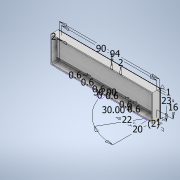
# Autodesk Inventor part: sdm_finger_eit_chamber_mould_horizontal_e_holes_v2
Saved by Autodesk Inventor 2021 (Build 250183000, 183)
## iProperties
Created: 2021-05-26
Part Number: sdm_finger_eit_chamber_mould_horizontal_e_holes_v2
Material: Generic
Document SubType Name: Modeling
Designer: Charlie
Density: 1 g/cm^3
Appearance: Default
Author: Charlie
Autodesk Inventor part; units mm, degrees
ref_plane "YZ Plane" through (0, 0, 0) normal (1, 0, 0) x (0, 1, 0)
ref_plane "XZ Plane" through (0, 0, 0) normal (0, 1, 0) x (-1, 0, 0)
ref_plane "XY Plane" through (0, 0, 0) normal (0, 0, 1) x (1, 0, 0)
sketch "Sketch2" plane through (0, 0, 0) normal (0, 0, 1) x (1, 0, 0)
  line L0 (-46, 11.5) -> (46, 11.5)
  line L1 (47, 10.5) -> (47, -10.5)
  line L2 (46, -11.5) -> (-46, -11.5)
  line L3 (-47, -10.5) -> (-47, 10.5)
  line L4 (-47, 11.5) -> (47, -11.5) construction
  line L5 (47, 11.5) -> (-47, -11.5) construction
  line L6 (48, 12.5) -> (-48, 12.5)
  line L7 (-48, 12.5) -> (-48, -12.5)
  line L8 (-48, -12.5) -> (48, -12.5)
  line L9 (48, -12.5) -> (48, 12.5)
  arc A0 (47, 10.5) -> (46, 11.5) centre (46, 10.5) ccw
  arc A1 (46, -11.5) -> (47, -10.5) centre (46, -10.5) ccw
  arc A2 (-47, -10.5) -> (-46, -11.5) centre (-46, -10.5) ccw
  arc A3 (-46, 11.5) -> (-47, 10.5) centre (-46, 10.5) ccw
  line L10 (-45, -6.5) -> (45, -6.5)
  line L11 (45, -6.5) -> (45, 9.5)
  line L12 (45, 9.5) -> (-45, 9.5)
  line L13 (-45, 9.5) -> (-45, -6.5)
  point P0 (0, 0)
  point P1 (0, 1.6851)
  dimension "d0" = 94
  dimension "d1" = 23
  dimension "d3" = 1
  dimension "d10" = 1
  dimension "d84" = 90
  dimension "d85" = 16
  dimension "d86" = 2
  dimension "d87" = 2
  dimension "d95" = 2
  constraints: 28 end point, 8 point on circle, 8 point on line, 8 tangent, 6 parallel, 4 centre point, 3 equal radius, 3 perpendicular, 2 horizontal, 2 midpoint, 3 other
  measures "d0" distance of L4.end L5.end
  measures "d1" distance of L5.start L4.end
  measures "d3" distance between parallel lines of L0 L6
  measures "d10" radius of A0
  measures "d84" distance of L12.end L11.end
  measures "d85" distance of L11.end L10.end
  measures "d86" distance between parallel lines of L0 L12
  measures "d87" distance between parallel lines of L3 L13
  measures "d95" distance between parallel lines of L1 L11
extrude "Extrusion1" add sketch "Sketch2" along normal blind 1 contours L0 A0 L1 A1 L2 A2 L3 A3 | L9 L8 L7 L6 | L13 L12 L11 L10
extrude "Extrusion2" add sketch "Sketch2" along normal blind 7 contours L9 L8 L7 L6
extrude "Extrusion3" add sketch "Sketch2" along normal blind 4 contours L13 L12 L11 L10
sketch "Sketch4" plane through (-48, -12.5, 0) normal (0, -1, 0) x (1, 0, 0)
  circle A0 centre (22.1132, 5) radius 0.5
  circle A1 centre (29.8868, 5) radius 0.5
  circle A2 centre (44.1132, 5) radius 0.5
  circle A3 centre (51.8842, 5) radius 0.5
  circle A4 centre (66.1132, 5) radius 0.5
  circle A5 centre (73.8868, 5) radius 0.5
  line L0 (0, 6) -> (96, 6)
  line L1 (96, 7) -> (0, 7) projected
  line L2 (22.1132, 2) -> (22.1132, 2)
  line L3 (22.6132, 2.5) -> (22.6132, 8)
  line L4 (22.6132, 8) -> (21.6132, 8)
  line L5 (21.6132, 8) -> (21.6132, 2.5)
  line L6 (21.6132, 2) -> (22.6132, 8) construction
  line L7 (22.6132, 2) -> (21.6132, 8) construction
  line L8 (29.8868, 2) -> (29.8868, 2)
  line L9 (30.3868, 2.5) -> (30.3868, 8)
  line L10 (30.3868, 8) -> (29.3868, 8)
  line L11 (29.3868, 8) -> (29.3868, 2.5)
  line L12 (29.3868, 2) -> (30.3868, 8) construction
  line L13 (30.3868, 2) -> (29.3868, 8) construction
  line L14 (44.1132, 2) -> (44.1132, 2)
  line L15 (44.6132, 2.5) -> (44.6132, 8)
  line L16 (44.6132, 8) -> (43.6132, 8)
  line L17 (43.6132, 8) -> (43.6132, 2.5)
  line L18 (43.6132, 2) -> (44.6132, 8) construction
  line L19 (44.6132, 2) -> (43.6132, 8) construction
  line L20 (51.8842, 2) -> (51.8842, 2)
  line L21 (52.3842, 2.5) -> (52.3842, 8)
  line L22 (52.3842, 8) -> (51.3842, 8)
  line L23 (51.3842, 8) -> (51.3842, 2.5)
  line L24 (51.3842, 2) -> (52.3842, 8) construction
  line L25 (52.3842, 2) -> (51.3842, 8) construction
  line L26 (66.1132, 2) -> (66.1132, 2)
  line L27 (65.6132, 2.5) -> (65.6132, 8)
  line L28 (65.6132, 8) -> (66.6132, 8)
  line L29 (66.6132, 8) -> (66.6132, 2.5)
  line L30 (66.6132, 2) -> (65.6132, 8) construction
  line L31 (65.6132, 2) -> (66.6132, 8) construction
  line L32 (73.8868, 2) -> (73.8868, 2)
  line L33 (73.3868, 2.5) -> (73.3868, 8)
  line L34 (73.3868, 8) -> (74.3868, 8)
  line L35 (74.3868, 8) -> (74.3868, 2.5)
  line L36 (74.3868, 2) -> (73.3868, 8) construction
  line L37 (73.3868, 2) -> (74.3868, 8) construction
  arc A6 (21.6132, 2.5) -> (22.1132, 2) centre (22.1132, 2.5) ccw
  arc A7 (22.1132, 2) -> (22.6132, 2.5) centre (22.1132, 2.5) ccw
  arc A8 (29.3868, 2.5) -> (29.8868, 2) centre (29.8868, 2.5) ccw
  arc A9 (29.8868, 2) -> (30.3868, 2.5) centre (29.8868, 2.5) ccw
  arc A10 (43.6132, 2.5) -> (44.1132, 2) centre (44.1132, 2.5) ccw
  arc A11 (44.1132, 2) -> (44.6132, 2.5) centre (44.1132, 2.5) ccw
  arc A12 (51.3842, 2.5) -> (51.8842, 2) centre (51.8842, 2.5) ccw
  arc A13 (51.8842, 2) -> (52.3842, 2.5) centre (51.8842, 2.5) ccw
  arc A14 (65.6132, 2.5) -> (66.1132, 2) centre (66.1132, 2.5) ccw
  arc A15 (66.1132, 2) -> (66.6132, 2.5) centre (66.1132, 2.5) ccw
  arc A16 (73.3868, 2.5) -> (73.8868, 2) centre (73.8868, 2.5) ccw
  arc A17 (73.8868, 2) -> (74.3868, 2.5) centre (73.8868, 2.5) ccw
  point P0 (96, 0)
  point P1 (69, 6)
  point P2 (71, 6)
  point P3 (49, 6)
  point P4 (47, 6)
  point P5 (27, 6)
  point P6 (25, 6)
  point P7 (73.8868, 2)
  point P8 (66.1132, 2)
  point P9 (51.8842, 2)
  point P10 (44.1132, 2)
  point P11 (29.8868, 2)
  point P12 (22.1132, 2)
  dimension "d59" = 1
  dimension "d60" = 1
  dimension "d61" = 1
  dimension "d62" = 1
  dimension "d63" = 1
  dimension "d64" = 1
  dimension "d65" = 1
  dimension "d66" = 6
  dimension "d67" = 1
  dimension "d68" = 6
  dimension "d69" = 1
  dimension "d70" = 6
  dimension "d71" = 1
  dimension "d72" = 6
  dimension "d73" = 1
  dimension "d74" = 6
  dimension "d75" = 1
  dimension "d76" = 6
  dimension "d81" = 0.5
  constraints: 74 end point, 24 point on circle, 24 point on line, 24 tangent, 18 centre point, 12 midpoint, 12 parallel, 11 equal radius, 6 horizontal, 6 perpendicular
  measures "d59" diameter of A0
  measures "d60" diameter of A1
  measures "d61" diameter of A2
  measures "d62" diameter of A3
  measures "d63" diameter of A4
  measures "d64" diameter of A5
  measures "d65" distance of L4.end L3.end
  measures "d66" distance of L3.end L7.start
  measures "d67" distance of L10.end L9.end
  measures "d68" distance of L9.end L13.start
  measures "d69" distance of L16.end L15.end
  measures "d70" distance of L15.end L19.start
  measures "d71" distance of L22.end L21.end
  measures "d72" distance of L21.end L25.start
  measures "d73" distance of L27.end L28.end
  measures "d74" distance of L31.start L27.end
  measures "d75" distance of L33.end L34.end
  measures "d76" distance of L37.start L33.end
  measures "d81" radius of A6
sketch "Sketch3" plane through (0, -12.5, 4) normal (0, -1, 0) x (1, 0, 0)
  line L0 (-53.1158, -2.5) -> (46.8842, -2.5) construction
  line L1 (43, -1.5) -> (23, -1.5) construction
  line L2 (23, -1.5) -> (23, 3.5) construction
  line L3 (23, 3.5) -> (43, 3.5) construction
  line L4 (43, 3.5) -> (43, -1.5) construction
  line L5 (23, -1.5) -> (23, 3.7137) construction
  line L6 (43, -1.5) -> (40.1132, 3.5) construction
  line L7 (46.8842, -2.5) -> (46.8842, 3.2735) construction
  line L8 (23, -1.5) -> (25.8868, 3.5) construction
  line L9 (23, -1.5) -> (23, 3.1279) construction
  line L10 (21, -1.5) -> (18.1132, 3.5) construction
  line L11 (1, 3.5) -> (21, 3.5) construction
  line L12 (1, -1.5) -> (3.8868, 3.5) construction
  line L13 (-1, -1.5) -> (-3.8868, 3.5) construction
  line L14 (-21, 3.5) -> (-1, 3.5) construction
  line L15 (-21, -1.5) -> (-18.1132, 3.5) construction
  line L16 (-23, -1.5) -> (-25.8868, 3.5) construction
  line L17 (-43, 3.5) -> (-23, 3.5) construction
  line L18 (-43, -1.5) -> (-40.1132, 3.5) construction
  line L19 (43, 3.5) -> (-43, 3.5) construction
  line L20 (0, 3.5) -> (0, 3.5) construction
  circle A0 centre (-25.8868, -1.5) radius 0.3
  circle A1 centre (-18.1132, -1.5) radius 0.3
  circle A2 centre (-3.8868, -1.5) radius 0.3
  circle A3 centre (3.8842, -1.5) radius 0.3
  circle A4 centre (18.1132, -1.5) radius 0.3
  circle A5 centre (25.8868, -1.5) radius 0.3
  line L21 (-45, 0) -> (-45, 0) projected
  line L22 (45, 0) -> (45, 0) projected
  line L23 (-48, -4) -> (-48, -4) projected
  line L24 (-48, -1.5) -> (48, -1.5)
  line L25 (48, -4) -> (48, -4) projected
  line L26 (48, -4) -> (48, 3) projected
  point P0 (3.8842, 2.5)
  point P1 (25.8868, -1.5)
  point P2 (48, -0.5)
  dimension "d45" = 20
  dimension "d46" = 5
  dimension "d47" = 30
  dimension "d48" = 30
  dimension "d49" = 22
  dimension "d52" = 0
  dimension "d53" = 0.6
  dimension "d54" = 0.6
  dimension "d55" = 0.6
  dimension "d56" = 0.6
  dimension "d57" = 0.6
  dimension "d58" = 0.6
  dimension "d82" = 1
  constraints: 44 end point, 10 point on line, 6 centre point, 2 parallel, 1 collinear, 1 equal length, 1 horizontal, 1 midpoint, 1 perpendicular, 1 vertical
  measures "d45" distance of L4.end L2.start
  measures "d46" distance of L2.start L2.end
  measures "d47" angle of L7 L6
  measures "d48" angle of L8 L9
  measures "d49" distance of L4.end L10.start
  measures "d52" distance of L20.start L20.end
  measures "d53" diameter of A0
  measures "d54" diameter of A1
  measures "d55" diameter of A2
  measures "d56" diameter of A3
  measures "d57" diameter of A4
  measures "d58" diameter of A5
  measures "d82" distance of point (48, -0.5) point (48, -1.5)
extrude "Extrusion4" [suppressed]
extrude "Extrusion5" cut sketch "Sketch3" against normal blind 15
sketch "Sketch5" plane through (-48, -12.5, 0) normal (-1, 0, 0) x (0, 0, 1)
  line L0 (7, 1) -> (1, 1)
  line L1 (1, 1) -> (1, 6)
  line L2 (1, 6) -> (7, 6)
  line L3 (7, 6) -> (7, 1)
  circle A0 centre (2.5, 3.5) radius 0.75
  point P0 (0, 12.5)
  dimension "d88" = 1.5
  dimension "d89" = 1.5
  dimension "d90" = 2.5
  constraints: 8 end point, 2 parallel, 1 centre point, 1 horizontal, 1 perpendicular
  measures "d88" diameter of A0
  measures "d89" distance from line of A0.centre L1
  measures "d90" distance from line of L2 A0.centre
extrude "Extrusion6" cut sketch "Sketch5" against normal blind 2 contours A0
extrude "Extrusion7" add sketch "Sketch3" against normal blind 1
body "Solid1"
